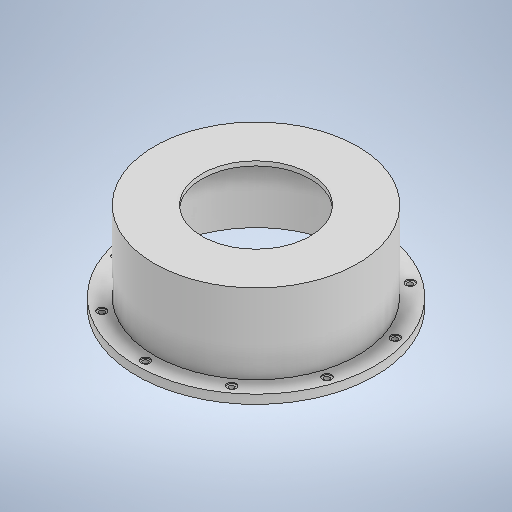
# Autodesk Inventor part: Vibrometer Housing
Saved by Autodesk Inventor 2026.2 (Build 302298000, 298)
## iProperties
Created: 2026-03-24
Part Number: Vibrometer Housing
Material: Generic
Document SubType Name: Modeling
Designer: mumin
Density: 1 g/cm^3
Appearance: Default
Author: mumin
Autodesk Inventor part; units mm, degrees
ref_plane "YZ Plane" through (0, 0, 0) normal (1, 0, 0) x (0, 1, 0)
ref_plane "XZ Plane" through (0, 0, 0) normal (0, 1, 0) x (-1, 0, 0)
ref_plane "XY Plane" through (0, 0, 0) normal (0, 0, 1) x (1, 0, 0)
sketch "Sketch1" plane through (0, 0, 0) normal (1, 0, 0) x (0, 1, 0)
  line L0 (0, 0) -> (120, 0)
  line L1 (100, -61.25) -> (95, -61.25)
  line L2 (95, -61.25) -> (95, -110)
  line L3 (95, -110) -> (0, -110)
  line L4 (0, -110) -> (0, -135)
  line L5 (0, -135) -> (10, -135)
  line L6 (10, -135) -> (10, -115)
  line L7 (10, -115) -> (100, -115)
  line L8 (100, -115) -> (100, -61.25)
  dimension "d1" = 270
  dimension "d2" = 220
  dimension "d3" = 230
  dimension "d4" = 122.5
  dimension "d5" = 10
  dimension "d6" = 5
  dimension "d7" = 100
  constraints: 18 end point, 7 perpendicular, 2 horizontal
  measures "d1" diameter of L5 L0
  measures "d2" diameter of L3 L0
  measures "d3" diameter of L7 L0
  measures "d4" diameter of L1 L0
  measures "d5" distance between parallel lines of L4 L6
  measures "d6" distance between parallel lines of L2 L8
  measures "d7" distance between parallel lines of L4 L8
revolve "Revolution1" add sketch "Sketch1" angle 360 about axis through (0, 0, 0) along (0, 1, 0)
sketch "Sketch2" plane through (0, 10, 0) normal (0, 1, 0) x (1, 0, 0)
  point P0 (0, 0)
  point P1 (0, 125)
  point P2 (-73.4732, 101.1271)
  point P3 (-118.8821, 38.6271)
  point P4 (-118.8821, -38.6271)
  point P5 (-73.4732, -101.1271)
  point P6 (0, -125)
  point P7 (73.4732, -101.1271)
  point P8 (118.8821, -38.6271)
  point P9 (118.8821, 38.6271)
  point P10 (73.4732, 101.1271)
  dimension "d9" = 125
  dimension "d12" = 360
  constraints: 11 other
  measures "d9" distance of point (0, 0) point (0, 125)
hole "Hole1" at (0, 10, -125) at (-73.4732, 10, -101.1271) at (-118.8821, 10, -38.6271) at (-118.8821, 10, 38.6271) at (-73.4732, 10, 101.1271) at (0, 10, 125) at (73.4732, 10, 101.1271) at (118.8821, 10, 38.6271) at (118.8821, 10, -38.6271) at (73.4732, 10, -101.1271) direction (0, -1, 0) diameter 5.9 end through all counterbore diameter 10.2 counterbore depth 1.2
body "Solid1"
